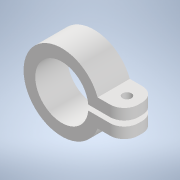
# Autodesk Inventor part: Cierre
Saved by Autodesk Inventor 2020 (Build 240168000, 168)
## iProperties
Created: 2022-03-24
Part Number: Cierre
Material: Genérico
Document SubType Name: Modeling
Designer: aarco
Density: 1 g/cm^3
Appearance: Valor por defecto
Author: aarco
Autodesk Inventor part; units mm, degrees
ref_plane "YZ Plane" through (0, 0, 0) normal (1, 0, 0) x (0, 1, 0)
ref_plane "XZ Plane" through (0, 0, 0) normal (0, 1, 0) x (-1, 0, 0)
ref_plane "XY Plane" through (0, 0, 0) normal (0, 0, 1) x (1, 0, 0)
sketch "Boceto1" plane through (0, 0, 0) normal (0, 0, 1) x (1, 0, 0)
  circle A0 centre (0, -3.2) radius 3.2 projected
  circle A1 centre (0, -3.2) radius 6.5 projected
  circle A2 centre (0, -3.2) radius 9.5
  circle A3 centre (0, -3.2) radius 6.6
  line L0 (5.5183, 0.15) -> (15.5, 0.15)
  line L1 (15.5, 0.15) -> (15.5, -2.55)
  line L2 (15.5, -2.55) -> (5.5183, -2.55)
  line L3 (5.5183, -2.55) -> (5.5183, 0.15)
  line L4 (5.5183, -3.85) -> (15.5, -3.85)
  line L5 (15.5, -3.85) -> (15.5, -6.55)
  line L6 (15.5, -6.55) -> (5.5183, -6.55)
  line L7 (5.5183, -6.55) -> (5.5183, -3.85)
  line L8 (0, -3.2) -> (15.5144, -3.2)
  line L9 (9.5, -3.2) -> (9.5, 8.1404)
  arc A4 (9.2965, -1.2441) -> (-9.2965, -1.2441) centre (0, -3.2) ccw projected
  point P0 (0, 0)
  point P1 (8.8897, 0.15)
  point P2 (8.8897, -6.55)
  point P3 (6.4674, -3.85)
  point P4 (5.5702, -6.55)
  point P5 (5.6866, -6.55)
  point P6 (6.5679, -2.55)
  point P7 (6.5679, -3.85)
  dimension "d0" = 0.1
  dimension "d1" = 6
  dimension "d2" = 1.3
  dimension "d3" = 2.7
  constraints: 20 end point, 4 parallel, 3 horizontal, 2 centre point, 2 coincident, 2 perpendicular, 2 point on circle, 2 point on line, 1 collinear, 1 symmetric about line, 1 tangent, 1 vertical, 1 vertical alignment, 1 other
  measures "d0" radial gap between concentric circles of A3 A1
  measures "d1" distance between parallel lines of L1 L9
  measures "d2" distance between parallel lines of L4 L2
  measures "d3" distance between parallel lines of L0 L2
extrude "Extrusión1" add sketch "Boceto1" against normal blind 8 contours A3 L0 A2 L2 | L4 A2 L6 A3 | A3 L6 A2 L0 | A2 L0 L9 L2 | L4 L5 L6 A2 | L9 L0 L1 L2
sketch "Boceto2" plane through (8.8897, -6.55, 0) normal (0, -1, 0) x (1, 0, 0)
  line L0 (0, 0) -> (6.6103, 0) projected
  line L1 (0, 0) -> (0, -8) projected
  line L2 (6.6103, -8) -> (0, -8) projected
  line L3 (6.6103, 0) -> (6.6103, -8) projected
  line L4 (0, 0) -> (0, -8) projected
  line L5 (6.6103, 0) -> (6.6103, -8) projected
  line L6 (0, 0) -> (6.6103, -8)
  line L7 (1.3051, -2.8453) -> (3.3051, -1.6906)
  line L8 (3.3051, -1.6906) -> (5.3051, -2.8453)
  line L9 (5.3051, -2.8453) -> (5.3051, -5.1547)
  line L10 (5.3051, -5.1547) -> (3.3051, -6.3094)
  line L11 (3.3051, -6.3094) -> (1.3051, -5.1547)
  line L12 (1.3051, -5.1547) -> (1.3051, -2.8453)
  point P0 (-8.8897, 0)
  point P1 (3.3051, -4)
  dimension "d6" = 4
  constraints: 14 end point, 1 midpoint, 1 vertical, 13 other
  measures "d6" distance between parallel lines of L12 L9
extrude "Extrusión2" cut sketch "Boceto2" against normal blind 1.35 contours L7 L8 L9 L10 L6 | L6 L10 L11 L12 L7
sketch "Boceto3" plane through (8.8897, -5.2, 0) normal (0, -1, 0) x (1, 0, 0)
  line L0 (3.3051, -6.3094) -> (1.3051, -5.1547) projected
  line L1 (5.3051, -2.8453) -> (1.3051, -5.1547)
  circle A0 centre (3.3051, -4) radius 1.1
  point P0 (-8.8897, 0)
  dimension "d9" = 2.2
  constraints: 2 end point, 1 centre point, 1 midpoint
  measures "d9" diameter of A0
extrude "Extrusión3" cut sketch "Boceto3" against normal through all
fillet "Empalme1" radius 3.5 4 edges at (15.5, -1.2, -8) (15.5, -5.2, -8) (15.5, -5.2, 0) (15.5, -1.2, 0)
